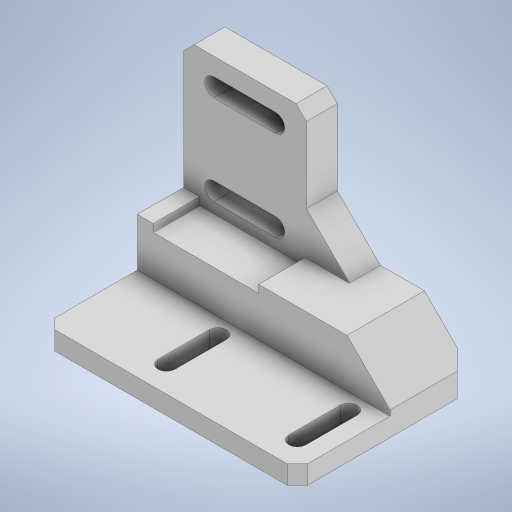
# Autodesk Inventor part: Motor Mount v2
Saved by Autodesk Inventor 2024 (Build 280153020, 153B)
## iProperties
Created: 2024-02-12
Part Number: Motor Mount v2
Material: Generic
Document SubType Name: Modeling
Designer: scottst
Density: 1 g/cm^3
Appearance: Default
Author: scottst
Autodesk Inventor part; units mm, degrees
ref_plane "YZ Plane" through (0, 0, 0) normal (1, 0, 0) x (0, 1, 0)
ref_plane "XZ Plane" through (0, 0, 0) normal (0, 1, 0) x (-1, 0, 0)
ref_plane "XY Plane" through (0, 0, 0) normal (0, 0, 1) x (1, 0, 0)
sketch "Sketch1" plane through (0, 0, 0) normal (1, 0, 0) x (0, 1, 0)
  line L0 (0, 0) -> (13, 0)
  line L1 (13, 0) -> (13, -27)
  line L2 (13, -27) -> (0, -27)
  line L3 (0, -27) -> (0, 0)
  dimension "d0" = 13
  dimension "d1" = 27
  constraints: 8 end point, 2 parallel, 1 horizontal, 1 perpendicular
  measures "d0" distance of L1.end L2.end
  measures "d1" distance of L0.end L1.end
extrude "Extrusion1" add sketch "Sketch1" along normal blind 40
sketch "Sketch2" plane through (40, 0, 0) normal (1, 0, 0) x (0, 0, -1)
  line L0 (27, 0) -> (27, 13) projected
  line L1 (27, 0) -> (33, 0)
  line L2 (33, 0) -> (33, 38)
  line L3 (33, 38) -> (27, 38)
  line L4 (27, 38) -> (27, 0)
  point P0 (0, 0)
  dimension "d4" = 6
  dimension "d5" = 38
  constraints: 8 end point, 2 parallel, 1 horizontal, 1 perpendicular
  measures "d4" distance of L3.end L2.end
  measures "d5" distance of L2.end L1.end
extrude "Extrusion2" add sketch "Sketch2" against normal blind 40
sketch "Sketch3" plane through (0, 13, 0) normal (0, 1, 0) x (1, 0, 0)
  line L0 (40, 27) -> (40, 0) construction
  line L1 (40, 0) -> (35, 0) construction
  line L2 (0, 0) -> (40, 0) construction
  line L3 (35, 0) -> (35, 5) construction
  line L4 (35, 5) -> (35, 15) construction
  line L5 (35, 5) -> (9.6, 5) construction
  line L6 (35, 5) -> (35, 15) construction
  line L7 (36.65, 5) -> (36.65, 15)
  line L8 (33.35, 15) -> (33.35, 5)
  arc A0 (33.35, 5) -> (36.65, 5) centre (35, 5) ccw
  arc A1 (36.65, 15) -> (33.35, 15) centre (35, 15) ccw
  line L9 (9.6, 0) -> (9.6, 5) construction
  line L10 (9.6, 5) -> (9.6, 15) construction
  line L11 (9.6, 5) -> (-15.8, 5) construction
  line L12 (9.6, 5) -> (9.6, 15) construction
  line L13 (11.25, 5) -> (11.25, 15)
  line L14 (7.95, 15) -> (7.95, 5)
  arc A2 (7.95, 5) -> (11.25, 5) centre (9.6, 5) ccw
  arc A3 (11.25, 15) -> (7.95, 15) centre (9.6, 15) ccw
  point P0 (35, 10)
  point P1 (9.6, 10)
  dimension "d8" = 5
  dimension "d9" = 5
  dimension "d10" = 10
  dimension "d11" = 25.4
  dimension "d12" = 3.3
  dimension "d13" = 5
  dimension "d14" = 10
  dimension "d15" = 25.4
  dimension "d16" = 3.3
  constraints: 30 end point, 8 point on circle, 8 tangent, 4 centre point, 4 equal length, 3 point on line, 2 horizontal, 2 midpoint, 1 perpendicular, 1 other
  measures "d8" distance of L0.end L1.end
  measures "d9" distance of L1.end L3.end
  measures "d10" distance of L3.end L4.end
  measures "d11" distance of L3.end L5.end
  measures "d12" diameter of A1
  measures "d13" distance of L9.start L9.end
  measures "d14" distance of L9.end L10.end
  measures "d15" distance of L9.end L11.end
  measures "d16" diameter of A3
extrude "Extrusion3" cut sketch "Sketch3" against normal blind 40
sketch "Sketch4" plane through (0, 13, 0) normal (0, 1, 0) x (1, 0, 0)
  point P0 (0, 0)
sketch "Sketch7" plane through (40, 13, -27) normal (0, 0, 1) x (1, 0, 0)
  line L0 (0, 25) -> (0, 0) projected
  line L1 (-40, 0) -> (0, 0) projected
  line L2 (0, 25) -> (-20, 25)
  line L3 (-20, 25) -> (-20, 0)
  line L4 (-20, 0) -> (0, 0)
  line L5 (0, 0) -> (0, 25)
  point P0 (-40, -13)
  constraints: 8 end point, 2 parallel, 1 horizontal, 1 midpoint, 1 perpendicular
extrude "Extrusion6" cut sketch "Sketch7" against normal blind 45.275
sketch "Sketch9" plane through (0, 0, 0) normal (-1, 0, 0) x (0, 0, 1)
  line L0 (0, 0) -> (0, 3.6) construction
  line L1 (0, 13) -> (0, 0) construction
  line L2 (0, 3.6) -> (-18, 3.6)
  line L3 (-18, 3.6) -> (-18, 13)
  line L4 (-18, 13) -> (0, 13)
  line L5 (0, 13) -> (0, 3.6)
  dimension "d58" = 3.6
  dimension "d59" = 18
  constraints: 10 end point, 2 parallel, 1 horizontal, 1 perpendicular, 1 point on line
  measures "d58" distance of L0.start L0.end
  measures "d59" distance of L3.end L4.end
extrude "Extrusion8" cut sketch "Sketch9" against normal blind 50.325
sketch "Sketch10" plane through (40, 0, -33) normal (0, 0, -1) x (-1, 0, 0)
  point P0 (40, 0)
sketch "Sketch8" plane through (0, 13, -27) normal (0, 1, 0) x (1, 0, 0)
  line L0 (0, 0) -> (20, 0) construction
  line L1 (0, 0) -> (2.5, 0) construction
  line L2 (2.5, 0) -> (14.5, 0)
  line L3 (14.5, 0) -> (14.5, -10)
  line L4 (14.5, -10) -> (2.5, -10)
  line L5 (2.5, -10) -> (2.5, 0)
  point P0 (0, -27)
  point P1 (26.7625, 0)
  dimension "d53" = 2.5
  dimension "d54" = 12
  dimension "d55" = 10
  constraints: 10 end point, 2 parallel, 1 horizontal, 1 perpendicular, 1 point on line
  measures "d53" distance of L0.start L1.end
  measures "d54" distance of L3.end L4.end
  measures "d55" distance of L2.end L3.end
extrude "Extrusion7" cut sketch "Sketch8" against normal blind 1.5
sketch "Sketch11" plane through (0, 0, 0) normal (-1, 0, 0) x (0, 0, 1)
  line L0 (0, 3.6) -> (-18, 3.6) projected
  line L1 (-18, 3.6) -> (-18, 13) projected
  line L2 (-27, 13) -> (-18, 13) projected
  line L3 (-27, 13) -> (-27, 38) projected
  line L4 (-27, 38) -> (-33, 38) projected
  line L5 (-33, 38) -> (-33, 0) projected
  line L6 (0, 0) -> (-33, 0) projected
  line L7 (0, 3.6) -> (0, 0) projected
extrude "Extrusion9" add sketch "Sketch11" along normal blind 9.05
sketch "Sketch6" plane through (40, 13, -27) normal (0, 0, 1) x (1, 0, 0)
  line L0 (-40, 0) -> (0, 0) construction
  line L1 (-47.2016, 0) -> (-47.2016, 2.3001) construction
  line L2 (-40, 25) -> (-40, -13) construction
  line L3 (-47.2016, 2.3001) -> (-13.7954, 2.3001) construction
  line L4 (-47.2016, 2.3001) -> (-47.2016, 19.8001) construction
  line L5 (-47.2016, 19.8001) -> (-14.7386, 19.8001) construction
  line L6 (-47.2016, 2.3001) -> (-43.2016, 2.3001) construction
  line L7 (-43.2016, 2.3001) -> (-43.2016, 19.8001) construction
  line L8 (-43.2016, 19.8001) -> (-31.2016, 19.8001) construction
  line L9 (-43.2016, 2.3001) -> (-31.2016, 2.3001) construction
  line L10 (-43.2016, 19.8001) -> (-31.2016, 19.8001) construction
  line L11 (-43.2016, 18.0501) -> (-31.2016, 18.0501)
  line L12 (-31.2016, 21.5501) -> (-43.2016, 21.5501)
  arc A0 (-43.2016, 21.5501) -> (-43.2016, 18.0501) centre (-43.2016, 19.8001) ccw
  arc A1 (-31.2016, 18.0501) -> (-31.2016, 21.5501) centre (-31.2016, 19.8001) ccw
  line L13 (-43.2016, 2.3001) -> (-31.2016, 2.3001) construction
  line L14 (-43.2016, 0.5501) -> (-31.2016, 0.5501)
  line L15 (-31.2016, 4.0501) -> (-43.2016, 4.0501)
  arc A2 (-43.2016, 4.0501) -> (-43.2016, 0.5501) centre (-43.2016, 2.3001) ccw
  arc A3 (-31.2016, 0.5501) -> (-31.2016, 4.0501) centre (-31.2016, 2.3001) ccw
  point P0 (-37.2016, 19.8001)
  point P1 (-37.2016, 2.3001)
  dimension "d28" = 7.56
  dimension "d29" = 17.5
  dimension "d30" = 4
  dimension "d31" = 12
  dimension "d32" = 12
  dimension "d33" = 3.5
  dimension "d34" = 3.5
  constraints: 32 end point, 8 point on circle, 8 tangent, 4 centre point, 4 point on line, 3 perpendicular, 2 collinear, 2 midpoint, 2 parallel
  measures "d28" distance of L0.start L1.end
  measures "d29" distance of L1.end L4.end
  measures "d30" distance of L1.end L6.end
  measures "d31" distance of L7.end L8.end
  measures "d32" distance of L6.end L9.end
  measures "d33" diameter of A1
  measures "d34" diameter of A3
extrude "Extrusion5" cut sketch "Sketch6" against normal blind 35.6875
sketch "Sketch13" plane through (2.5, 13, -18) normal (0, 1, 0) x (1, 0, 0)
  line L0 (-11.55, 0) -> (37.5, 0) projected
  line L1 (6.2984, 9) -> (-5.7016, 9) projected
  line L2 (-8.4479, 0) -> (0.0285, 0)
  line L3 (0.0285, 0) -> (0.0285, 9)
  line L4 (0.0285, 9) -> (-8.4479, 9)
  line L5 (-8.4479, 9) -> (-8.4479, 0)
  point P0 (-2.5, -18)
  point P1 (5.45, 0)
  point P2 (0.0285, 0)
  point P3 (-5.7016, 9)
  constraints: 8 end point, 2 parallel, 2 point on line, 1 horizontal, 1 perpendicular
extrude "Extrusion10" cut sketch "Sketch13" against normal up to surface (1.5 mm away)
chamfer "Chamfer5" distance 8.35 angle 45 1 edges at (40, 13, -25.5)
sketch "Sketch14" plane through (20, 13, -27) normal (1, 0, 0) x (0, 0, -1)
  line L0 (6, 25) -> (6, 0) projected
  line L1 (0, 25) -> (6, 25) projected
  line L2 (0, 0) -> (0, 25) projected
  line L3 (0, 0) -> (6, 0) projected
  point P0 (-27, -13)
extrude "Extrusion11" cut sketch "Sketch14" against normal blind 5.2375
chamfer "Chamfer6" distance 8.35 angle 45 1 edges at (14.7625, 13, -30)
chamfer "Chamfer7" distance 2 angle 45 2 edges at (14.7625, 38, -30) (-9.05, 38, -30)
chamfer "Chamfer8" distance 2 angle 45 4 edges at (40, 1.8, 0) (-9.05, 1.8, 0) (40, 2.325, -33) (-9.05, 18, -33)
body "Solid1"
